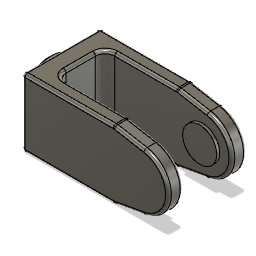
Link4 (Autodesk Fusion 360 design; units mm, degrees)
Autodesk Fusion 360 part; units mm, degrees
sketch "Sketch1" plane through (0, 0, 0) normal (0, 0, 1) x (1, 0, 0)
  line L0 (0, 0) -> (94.2683, 0)
  line L1 (94.2683, 0) -> (125.2094, 5.4558)
  arc A0 (125.2094, 5.4558) -> (125.2094, 64.5442) centre (120, 35) ccw
  line L2 (125.2094, 64.5442) -> (94.2683, 70)
  line L3 (94.2683, 70) -> (0, 70)
  line L4 (0, 70) -> (0, 0)
  dimension "d1" = 70
  dimension "d2" = 30
  dimension "d3" = 170
  dimension "d4" = 120
  constraint coincident L0.start L4.end
  constraint horizontal L0
  constraint tangent L1 A0
  constraint tangent A0 L2
  constraint horizontal L3
  constraint perpendicular L0 L4
  constraint equal L1 L2
  constraint equal L0 L3
  measures "d1" distance of L0 L3
  measures "d2" radius of A0
  measures "d3" angle of L0 L1
  measures "d4" horizontal distance of L0.start A0.centre
extrude "Extrude1" add sketch "Sketch1" along normal mid plane 80
sketch "Sketch2" plane through (0, 70, 0) normal (0, 1, 0) x (-1, 0, 0)
  line L0 (0, -40) -> (0, 40)
  line L1 (0, 40) -> (-94.2683, 40)
  line L2 (-94.2683, 40) -> (-94.2683, -40)
  line L3 (-94.2683, -40) -> (0, -40)
  line L4 (-20, -25) -> (-190, -25)
  line L5 (-190, -25) -> (-190, 25)
  line L6 (-190, 25) -> (-20, 25)
  line L7 (-20, 25) -> (-20, -25)
  dimension "d7" = 15
  dimension "d8" = 15
  dimension "d9" = 20
  dimension "d10" = 170
  constraint horizontal L4
  constraint vertical L5
  constraint horizontal L6
  constraint vertical L7
  measures "d7" distance of L3 L4
  measures "d8" distance of L1 L6
  measures "d9" distance of L0 L7
  measures "d10" distance of L5.end L6.end
extrude "Extrude2" cut sketch "Sketch2" against normal through all contours L2 L4 L5 L6 | L2 L4 L6 L7
sketch "Sketch3" plane through (0, 0, -25) normal (0, 0, 1) x (1, 0, 0)
  line L0 (20, 0) -> (94.2683, 0)
  line L1 (94.2683, 0) -> (125.2094, 5.4558)
  arc A0 (125.2094, 5.4558) -> (125.2094, 64.5442) centre (120, 35) ccw
  line L2 (125.2094, 64.5442) -> (94.2683, 70)
  line L3 (94.2683, 70) -> (20, 70)
  line L4 (20, 70) -> (20, 0)
  circle A1 centre (120, 35) radius 17.5
  dimension "d12" = 35
  constraint concentric A0 A1
  measures "d12" diameter of A1
extrude "Extrude3" add sketch "Sketch3" along normal blind 3 contours A1
mirror "Mirror1" about plane through (0, 0, 0) normal (0, 0, 1) of "Extrude3"
sketch "Sketch4" plane through (0, 0, 0) normal (-1, 0, 0) x (0, 0, 1)
  line L0 (-40, 0) -> (40, 0)
  line L1 (40, 0) -> (40, 70)
  line L2 (40, 70) -> (-40, 70)
  line L3 (-40, 70) -> (-40, 0)
  circle A0 centre (0, 35) radius 25
  line L4 (0, 35) -> (-40, 35) construction
  line L5 (0, 35) -> (0, 0) construction
  dimension "d16" = 50
  constraint coincident A0.centre L4.start
  constraint midpoint L3 L4.end
  constraint perpendicular L3 L4
  constraint coincident L5.end origin
  constraint perpendicular L0 L5
  measures "d16" diameter of A0
extrude "Extrude4" add sketch "Sketch4" along normal blind 10 contours A0
sketch "Sketch5" plane through (-10, 0, 0) normal (-1, 0, 0) x (0, 0, 1)
  circle A0 centre (0, 35) radius 25
  circle A1 centre (0, 35) radius 22
  dimension "d19" = -3
extrude "Extrude5" add sketch "Sketch5" along normal blind 3 contours A1
fillet "Fillet1" radius 10 6 edges at (20, 35, 25) (20, 35, -25) (94.2683, 70, 32.5) (94.2683, 70, -32.5) (94.2683, 0, 32.5) (94.2683, 0, -32.5)
fillet "Fillet2" radius 3 39 edges at (46.6967, 0, 40) (94.2649, 0.0381, 40) (110.1696, 2.8038, 40) (150, 35, 40) (110.1696, 67.1962, 40) (94.2649, 69.9619, 40) (46.6967, 70, 40) (46.6967, 70, -40) (94.2649, 69.9619, -40) (110.1696, 67.1962, -40) (150, 35, -40) (110.1696, 2.8038, -40) (94.2649, 0.0381, -40) (46.6967, 0, -40) (0, 70, 0) (0, 35, 40) (0, 35, -40) (0, 0, 0) (0, 44.0404, -23.3082) (22.9289, 70, 22.0711) (20, 70, 0) (22.9289, 70, -22.0711) (61.6967, 70, -25) (94.2649, 69.9619, -25) (110.1696, 67.1962, -25) (150, 35, -25) (110.1696, 2.8038, -25) (94.2649, 0.0381, -25) (61.6967, 0, -25) (22.9289, 0, -22.0711) (20, 0, 0) (22.9289, 0, 22.0711) (61.6967, 0, 25) (94.2649, 0.0381, 25) (110.1696, 2.8038, 25) (150, 35, 25) (110.1696, 67.1962, 25) (94.2649, 69.9619, 25) (61.6967, 70, 25)
